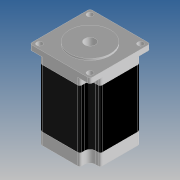
# Autodesk Inventor part: Motor
Saved by Autodesk Inventor 2017 (Build 210142000, 142)
## iProperties
Part Number: Motor
Material: Genérico
Document SubType Name: Modeling
Designer: Leo
Density: 1 g/cm^3
Appearance: Valor por defecto
Author: Leo
Autodesk Inventor part; units mm, degrees
ref_plane "YZ Plane" through (0, 0, 0) normal (1, 0, 0) x (0, 1, 0)
ref_plane "XZ Plane" through (0, 0, 0) normal (0, 1, 0) x (-1, 0, 0)
ref_plane "XY Plane" through (0, 0, 0) normal (0, 0, 1) x (1, 0, 0)
sketch "Boceto1" plane through (0, 0, 0) normal (0, 0, 1) x (1, 0, 0)
  line L0 (-26, 28) -> (26, 28)
  line L1 (28, 26) -> (28, -26)
  line L2 (26, -28) -> (-26, -28)
  line L3 (-28, -26) -> (-28, 26)
  arc A0 (-26, 28) -> (-28, 26) centre (-26, 26) ccw
  arc A1 (28, 26) -> (26, 28) centre (26, 26) ccw
  arc A2 (26, -28) -> (28, -26) centre (26, -26) ccw
  arc A3 (-28, -26) -> (-26, -28) centre (-26, -26) ccw
  line L4 (-26, 26) -> (26, -26) construction
  line L5 (-26, -26) -> (26, 26) construction
  circle A4 centre (23.4406, 23.4406) radius 2.65
  circle A5 centre (23.4406, -23.4406) radius 2.65
  circle A6 centre (-23.4406, -23.4406) radius 2.65
  circle A7 centre (-23.4406, 23.4406) radius 2.65
  circle A8 centre (0, 0) radius 5
  point P0 (-28, 28)
  point P1 (-28, -28)
  dimension "d0" = 56
  dimension "d1" = 2
  dimension "d2" = 5.3
  dimension "d3" = 61
  dimension "d4" = 10
  constraints: 12 end point, 9 centre point, 8 point on circle, 8 point on line, 8 tangent, 6 equal radius, 2 coincident, 2 horizontal alignment, 2 parallel, 2 perpendicular, 2 vertical alignment, 1 horizontal, 1 midpoint
  measures "d0" distance of point (-28, -28) point (-28, 28)
  measures "d1" radius of A0
  measures "d2" diameter of A4
  measures "d4" diameter of A8
extrude "Extrusión1" add sketch "Boceto1" against normal blind 4.7
sketch "Boceto2" plane through (0, 0, -4.7) normal (0, 0, -1) x (-1, 0, 0)
  circle A0 centre (0, 0) radius 5 projected
  circle A1 centre (-23.4406, 23.4406) radius 2.65 construction
  circle A2 centre (23.4406, 23.4406) radius 2.65 construction
  circle A3 centre (23.4406, -23.4406) radius 2.65 construction
  circle A4 centre (-23.4406, -23.4406) radius 2.65 construction
  arc A5 (-23.4406, 18.5) -> (-18.5, 23.4406) centre (-23.4406, 23.4406) ccw
  arc A6 (18.5, 23.4406) -> (23.4406, 18.5) centre (23.4406, 23.4406) ccw
  arc A7 (23.4406, -18.5) -> (18.5, -23.4406) centre (23.4406, -23.4406) ccw
  arc A8 (-18.5, -23.4406) -> (-23.4406, -18.5) centre (-23.4406, -23.4406) ccw
  line L0 (-18.5, 23.4406) -> (-18.5, 28)
  line L1 (26, 28) -> (-26, 28) construction
  line L2 (18.5, 23.4406) -> (18.5, 28)
  line L3 (23.4406, 18.5) -> (28, 18.5)
  line L4 (28, -26) -> (28, 26) construction
  line L5 (23.4406, -18.5) -> (28, -18.5)
  line L6 (18.5, -23.4406) -> (18.5, -28)
  line L7 (-26, -28) -> (26, -28) construction
  line L8 (-18.5, -23.4406) -> (-18.5, -28)
  line L9 (-23.4406, -18.5) -> (-28, -18.5)
  line L10 (-28, 26) -> (-28, -26) construction
  line L11 (-23.4406, 18.5) -> (-28, 18.5)
  line L12 (-28, -18.5) -> (-28, 18.5)
  line L13 (-18.5, 28) -> (18.5, 28)
  line L14 (28, 18.5) -> (28, -18.5)
  line L15 (18.5, -28) -> (-18.5, -28)
  dimension "d7" = 37
  constraints: 24 end point, 8 point on circle, 8 point on line, 5 tangent, 4 centre point, 4 coincident, 4 perpendicular, 3 equal length, 3 equal radius, 3 parallel, 2 horizontal, 2 vertical, 1 collinear
  measures "d7" distance between parallel lines of L2 L0
extrude "Extrusión2" add sketch "Boceto2" along normal blind 71.3
sketch "Boceto3" plane through (0, 0, 0) normal (0, 0, 1) x (1, 0, 0)
  circle A0 centre (0, 0) radius 5 projected
  circle A1 centre (0, 0) radius 19
  dimension "d10" = 38
  constraints: 1 centre point, 1 coincident
  measures "d10" diameter of A1
extrude "Extrusión3" add sketch "Boceto3" along normal blind 1.6
fillet "Empalme1" radius 2 8 edges at (18.5, 28, -40.35) (28, 18.5, -40.35) (-18.5, 28, -40.35) (-28, 18.5, -40.35) (28, -18.5, -40.35) (18.5, -28, -40.35) (-18.5, -28, -40.35) (-28, -18.5, -40.35)
ref_plane "Plano de trabajo1" through (0, 0, -11) normal (0, 0, 1) x (1, 0, 0)
ref_plane "Plano de trabajo2" through (0, 0, -65) normal (0, 0, -1) x (-1, 0, 0)
split body "Dividir1" result two bodies by plane through (0, 0, -11) normal (0, 0, 1) first body at (-0.2009, 20.3212, -10.5)
split body "Dividir2" result two bodies by plane through (0, 0, -65) normal (0, 0, -1) bodies 3 first body at (-0.2009, 20.3212, -65.5)
